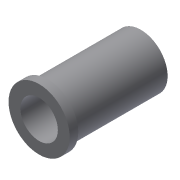
# Autodesk Inventor part: Bush bottomplate2
Saved by Autodesk Inventor 2022 (Build 260148000, 148)
## iProperties
Shininess: 64.0
Length Units: 11272
Angle Units: 11279
Time Units: 11290
Mass Units: 11286
Length Display Precision: 3
Angle Display Precision: 2
Compacted: True
Part Number: Bush bottomplate2
Document SubType Name: Modeling
Created: 2003-04-07
Designer: demo
Density: 1 g/cm^3
Material: Generic
Appearance: Default
Density: 0.0
Volumn: 0.0
Area: 0.0
PropertySet Name: Model Information
Control State: 0
Master: False
Checked Out: False
Author: demo
Autodesk Inventor part; units mm, degrees
ref_plane "YZ Plane" through (0, 0, 0) normal (1, 0, 0) x (0, 1, 0)
ref_plane "XZ Plane" through (0, 0, 0) normal (0, 1, 0) x (-1, 0, 0)
ref_plane "XY Plane" through (0, 0, 0) normal (0, 0, 1) x (1, 0, 0)
sketch "Sketch1" plane through (0, 0, 0) normal (0, 0, 1) x (1, 0, 0)
  circle A0 centre (-69.85, -69.85) radius 15.875 projected
  circle A1 centre (-69.85, -69.85) radius 18.1229
  dimension "d0" = 36.2458
  constraints: 1 centre point, 1 coincident, 1 concentric
  measures "d0" diameter of A1
extrude "Extrusion1" add sketch "Sketch1" along normal blind 5.08 contours A0 | A1
sketch "Sketch2" plane through (-69.85, -69.85, 0) normal (0, 0, -1) x (-1, 0, 0)
  circle A0 centre (0, 0) radius 18.1229 projected
  circle A1 centre (0, 0) radius 15.875
  dimension "d3" = 31.75
  constraints: 1 centre point, 1 coincident, 1 concentric
  measures "d3" diameter of A1
extrude "Extrusion2" add sketch "Sketch2" along normal blind 55.245 contours A1
sketch "Sketch3" plane through (-69.85, -69.85, 5.08) normal (0, 0, 1) x (1, 0, 0)
  circle A0 centre (0, 0) radius 18.1229 projected
  circle A1 centre (0, 0) radius 11.1125
  dimension "d6" = 22.225
  constraints: 1 centre point, 1 coincident, 1 concentric
  measures "d6" diameter of A1
extrude "Extrusion3" cut sketch "Sketch3" against normal through all contours A1
body "Solid1"
